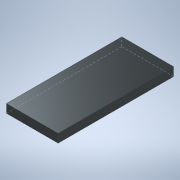
# Autodesk Inventor part: GateLatch
Saved by Autodesk Inventor 2020 (Build 240168000, 168)
## iProperties
Created: 2020-06-06
Part Number: GateLatch
Material: Iron, Cast
Document SubType Name: Modeling
Designer: user
Density: 7.15 g/cm^3
Appearance: Iron Gray
Author: user
Autodesk Inventor part; units mm, degrees
ref_plane "YZ Plane" through (0, 0, 0) normal (1, 0, 0) x (0, 1, 0)
ref_plane "XZ Plane" through (0, 0, 0) normal (0, 1, 0) x (-1, 0, 0)
ref_plane "XY Plane" through (0, 0, 0) normal (0, 0, 1) x (1, 0, 0)
sketch "Sketch1" plane through (0, 0, 0) normal (0, 1, 0) x (-1, 0, 0)
  line L0 (13.65, 29.9672) -> (-13.65, 29.9672)
  line L1 (-13.65, 29.9672) -> (-13.65, -30.9086)
  line L2 (-13.65, -30.9086) -> (13.65, -30.9086)
  line L3 (13.65, -30.9086) -> (13.65, 29.9672)
  point P0 (0, 0)
  dimension "d0" = 27.3
  constraints: 8 end point, 2 parallel, 1 horizontal, 1 perpendicular
  measures "d0" distance between parallel lines of L1 L3
extrude "Extrusion1" add sketch "Sketch1" along normal blind 4.48
body "Solid1"
